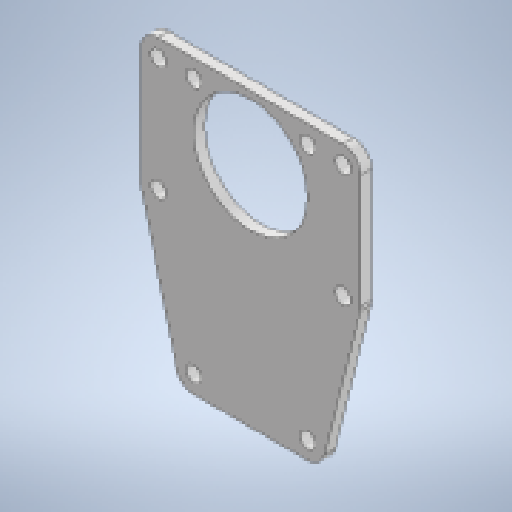
# Autodesk Inventor part: jouhansin_sita
Saved by Autodesk Inventor 2025.1 (Build 291241000, 241)
## iProperties
Created: 2024-09-01
Part Number: jouhansin_sita
Material: 一般
Document SubType Name: Modeling
Designer: right
Density: 1 g/cm^3
Appearance: 既定
Author: right
Autodesk Inventor part; units mm, degrees
ref_plane "YZ Plane" through (0, 0, 0) normal (1, 0, 0) x (0, 1, 0)
ref_plane "XZ Plane" through (0, 0, 0) normal (0, 1, 0) x (-1, 0, 0)
ref_plane "XY Plane" through (0, 0, 0) normal (0, 0, 1) x (1, 0, 0)
sketch "スケッチ1" plane through (0, 0, 0) normal (0, 0, 1) x (1, 0, 0)
  circle A0 centre (55.7151, -22.426) radius 1 projected
  circle A1 centre (55.7151, -6.426) radius 1.05 projected
  circle A2 centre (20.7151, -6.426) radius 1 projected
  circle A3 centre (4.7151, -6.426) radius 1.45 projected
  circle A4 centre (-30.2849, -22.426) radius 1 projected
  circle A5 centre (-30.2849, -6.426) radius 1.05 projected
  circle A6 centre (55.7151, -22.426) radius 1.1
  circle A7 centre (55.7151, -6.426) radius 1.1
  circle A8 centre (20.7151, -6.426) radius 1.1
  circle A9 centre (4.7151, -6.426) radius 1.1
  circle A10 centre (-30.2849, -6.426) radius 1.1
  circle A11 centre (-30.2849, -22.426) radius 1.1
  circle A12 centre (20.7151, -42.426) radius 1 projected
  circle A13 centre (4.7151, -42.426) radius 1 projected
  circle A14 centre (20.7151, -42.426) radius 1.1
  circle A15 centre (4.7151, -42.426) radius 1.1
  circle A16 centre (55.7151, -6.426) radius 2.5
  circle A17 centre (-30.2849, -6.426) radius 2.5
  circle A18 centre (-30.2849, -22.426) radius 2.5
  circle A19 centre (55.7151, -22.426) radius 2.5
  circle A20 centre (20.7151, -42.426) radius 2.5
  circle A21 centre (4.7151, -42.426) radius 2.5
  line L0 (21.9554, -44.5966) -> (56.9554, -24.5966)
  line L1 (58.2151, -22.426) -> (58.2151, -6.426)
  line L2 (55.7151, -3.926) -> (-30.2849, -3.926)
  line L3 (-32.7849, -6.426) -> (-32.7849, -22.426)
  line L4 (3.4747, -44.5966) -> (-31.5253, -24.5966)
  line L5 (20.7151, -44.926) -> (4.7151, -44.926)
  circle A22 centre (91.7151, -22.426) radius 1 projected
  circle A23 centre (91.7151, -22.426) radius 1.1
  circle A24 centre (-66.2849, -22.426) radius 1.05 projected
  circle A25 centre (-66.2849, -22.426) radius 1.1
  circle A26 centre (-66.2849, -22.426) radius 2.5
  circle A27 centre (91.7151, -22.426) radius 2.5
  line L6 (92.3929, -24.8324) -> (21.3929, -44.8324)
  line L7 (91.7151, -19.926) -> (55.7151, -19.926)
  line L8 (73.8937, -20.8546) -> (67.5365, -20.8546) projected
  line L9 (73.8937, -16.9974) -> (73.8937, -20.8546) projected
  line L10 (67.5365, -16.9974) -> (73.8937, -16.9974) projected
  line L11 (67.5365, -20.8546) -> (67.5365, -16.9974) projected
  line L12 (73.8937, -20.8546) -> (67.5365, -20.8546) projected
  line L13 (67.6151, -17.226) -> (73.6151, -17.226) projected
  line L14 (73.6151, -17.226) -> (73.6151, -20.726) projected
  line L15 (73.6151, -20.726) -> (67.6151, -20.726) projected
  line L16 (67.6151, -20.726) -> (67.6151, -17.226) projected
  line L17 (65.6151, -22.726) -> (75.6151, -22.726)
  line L18 (75.6151, -22.726) -> (75.6151, -15.226)
  line L19 (75.6151, -15.226) -> (65.6151, -15.226)
  line L20 (65.6151, -15.226) -> (65.6151, -22.726)
  line L21 (-66.9603, -24.833) -> (3.4747, -44.5966)
  line L22 (-30.2849, -19.926) -> (-66.2849, -19.926)
  line L23 (-48.4635, -20.8546) -> (-48.4635, -16.9974) projected
  line L24 (-28.7849, -24.426) -> (-67.7849, -24.426) projected
  arc A28 (-28.7849, -24.426) -> (-28.2849, -23.926) centre (-28.7849, -23.926) ccw projected
  line L25 (-28.2849, -4.926) -> (-28.2849, -23.926) projected
  arc A29 (-28.2849, -4.926) -> (-28.7849, -4.426) centre (-28.7849, -4.926) ccw projected
  line L26 (-67.7849, -4.426) -> (-28.7849, -4.426) projected
  arc A30 (-67.7849, -4.426) -> (-68.2849, -4.926) centre (-67.7849, -4.926) ccw projected
  line L27 (-68.2849, -23.926) -> (-68.2849, -4.926) projected
  arc A31 (-68.2849, -23.926) -> (-67.7849, -24.426) centre (-67.7849, -23.926) ccw projected
  line L28 (-48.4635, -7.9974) -> (-42.1063, -7.9974) projected
  line L29 (-42.1063, -7.9974) -> (-42.1063, -11.8546) projected
  line L30 (-42.1063, -11.8546) -> (-48.4635, -11.8546) projected
  line L31 (-48.4635, -11.8546) -> (-48.4635, -7.9974) projected
  circle A32 centre (-40.8849, -14.426) radius 1.1519 projected
  line L32 (-48.4635, -20.8546) -> (-48.4635, -16.9974) projected
  line L33 (-48.4635, -16.9974) -> (-42.1063, -16.9974) projected
  line L34 (-42.1063, -16.9974) -> (-42.1063, -20.8546) projected
  line L35 (-42.1063, -20.8546) -> (-48.4635, -20.8546) projected
  circle A33 centre (-66.2849, -6.426) radius 1.8131 projected
  circle A34 centre (-66.2849, -22.426) radius 1.8131 projected
  circle A35 centre (-30.2849, -6.426) radius 1.8131 projected
  circle A36 centre (-30.2849, -22.426) radius 1.8131 projected
  arc A37 (-59.7956, -8.176) -> (-59.7849, -20.676) centre (-59.7849, -14.426) ccw projected
  arc A38 (-60.0349, -7.926) -> (-59.7956, -8.1758) centre (-59.7849, -7.926) ccw projected
  line L36 (-60.0349, -7.926) -> (-60.0349, -6.176) projected
  arc A39 (-59.5349, -6.176) -> (-60.0349, -6.176) centre (-59.7849, -6.176) ccw projected
  line L37 (-59.5349, -6.176) -> (-59.5349, -7.926) projected
  arc A40 (-59.7849, -8.176) -> (-59.5349, -7.926) centre (-59.7849, -7.926) ccw projected
  arc A41 (-57.3931, -8.6518) -> (-59.7849, -8.176) centre (-59.7849, -14.426) ccw projected
  arc A42 (-57.5284, -8.3251) -> (-57.3931, -8.6518) centre (-57.2975, -8.4208) ccw projected
  line L38 (-57.5284, -8.3251) -> (-56.8587, -6.7083) projected
  arc A43 (-56.3968, -6.8997) -> (-56.8587, -6.7083) centre (-56.6278, -6.804) ccw projected
  line L39 (-56.3968, -6.8997) -> (-57.0665, -8.5165) projected
  arc A44 (-57.3931, -8.6518) -> (-57.0665, -8.5165) centre (-57.2975, -8.4208) ccw projected
  arc A45 (-55.3655, -10.0066) -> (-57.3931, -8.6518) centre (-59.7849, -14.426) ccw projected
  arc A46 (-55.3655, -9.653) -> (-55.3655, -10.0066) centre (-55.1887, -9.8298) ccw projected
  line L40 (-55.3655, -9.653) -> (-54.1281, -8.4156) projected
  arc A47 (-53.7745, -8.7692) -> (-54.1281, -8.4156) centre (-53.9513, -8.5924) ccw projected
  line L41 (-53.7745, -8.7692) -> (-55.0119, -10.0066) projected
  arc A48 (-55.3655, -10.0066) -> (-55.0119, -10.0066) centre (-55.1887, -9.8298) ccw projected
  arc A49 (-54.0107, -12.0342) -> (-55.3655, -10.0066) centre (-59.7849, -14.426) ccw projected
  arc A50 (-53.8754, -11.7076) -> (-54.0107, -12.0342) centre (-53.7797, -11.9386) ccw projected
  line L42 (-53.8754, -11.7076) -> (-52.2586, -11.0379) projected
  arc A51 (-52.0672, -11.4998) -> (-52.2586, -11.0379) centre (-52.1629, -11.2689) ccw projected
  line L43 (-52.0672, -11.4998) -> (-53.684, -12.1695) projected
  arc A52 (-54.0107, -12.0342) -> (-53.684, -12.1695) centre (-53.7797, -11.9386) ccw projected
  arc A53 (-53.5349, -14.426) -> (-54.0107, -12.0342) centre (-59.7849, -14.426) ccw projected
  arc A54 (-53.2849, -14.176) -> (-53.5349, -14.426) centre (-53.2849, -14.426) ccw projected
  line L44 (-53.2849, -14.176) -> (-51.5349, -14.176) projected
  arc A55 (-51.5349, -14.676) -> (-51.5349, -14.176) centre (-51.5349, -14.426) ccw projected
  line L45 (-51.5349, -14.676) -> (-53.2849, -14.676) projected
  arc A56 (-53.5349, -14.426) -> (-53.2849, -14.676) centre (-53.2849, -14.426) ccw projected
  arc A57 (-54.0107, -16.8178) -> (-53.5349, -14.426) centre (-59.7849, -14.426) ccw projected
  arc A58 (-53.684, -16.6825) -> (-54.0107, -16.8178) centre (-53.7797, -16.9134) ccw projected
  line L46 (-53.684, -16.6825) -> (-52.0672, -17.3522) projected
  arc A59 (-52.2586, -17.8141) -> (-52.0672, -17.3522) centre (-52.1629, -17.5831) ccw projected
  line L47 (-52.2586, -17.8141) -> (-53.8754, -17.1444) projected
  arc A60 (-54.0107, -16.8178) -> (-53.8754, -17.1444) centre (-53.7797, -16.9134) ccw projected
  arc A61 (-55.3655, -18.8454) -> (-54.0107, -16.8178) centre (-59.7849, -14.426) ccw projected
  arc A62 (-55.0119, -18.8454) -> (-55.3655, -18.8454) centre (-55.1887, -19.0222) ccw projected
  line L48 (-55.0119, -18.8454) -> (-53.7745, -20.0829) projected
  arc A63 (-54.1281, -20.4364) -> (-53.7745, -20.0829) centre (-53.9513, -20.2596) ccw projected
  line L49 (-54.1281, -20.4364) -> (-55.3655, -19.199) projected
  arc A64 (-55.3655, -18.8454) -> (-55.3655, -19.199) centre (-55.1887, -19.0222) ccw projected
  arc A65 (-57.3931, -20.2003) -> (-55.3655, -18.8454) centre (-59.7849, -14.426) ccw projected
  arc A66 (-57.0665, -20.3356) -> (-57.3931, -20.2003) centre (-57.2975, -20.4312) ccw projected
  line L50 (-57.0665, -20.3356) -> (-56.3968, -21.9523) projected
  arc A67 (-56.8587, -22.1437) -> (-56.3968, -21.9523) centre (-56.6278, -22.048) ccw projected
  line L51 (-56.8587, -22.1437) -> (-57.5284, -20.5269) projected
  arc A68 (-57.3931, -20.2003) -> (-57.5284, -20.5269) centre (-57.2975, -20.4312) ccw projected
  arc A69 (-59.7849, -20.676) -> (-57.3931, -20.2003) centre (-59.7849, -14.426) ccw projected
  arc A70 (-59.5349, -20.926) -> (-59.7849, -20.676) centre (-59.7849, -20.926) ccw projected
  line L52 (-59.5349, -20.926) -> (-59.5349, -22.676) projected
  arc A71 (-60.0349, -22.676) -> (-59.5349, -22.676) centre (-59.7849, -22.676) ccw projected
  line L53 (-60.0349, -22.676) -> (-60.0349, -20.926) projected
  arc A72 (-59.7849, -20.676) -> (-60.0349, -20.926) centre (-59.7849, -20.926) ccw projected
  line L54 (-50.4635, -22.8546) -> (-40.1063, -22.8546)
  line L55 (-40.1063, -22.8546) -> (-40.1063, -14.9974)
  line L56 (-40.1063, -14.9974) -> (-50.4635, -14.9974)
  line L57 (-50.4635, -22.8546) -> (-50.4635, -14.9974)
  circle A73 centre (-59.7849, -14.426) radius 8 projected
  circle A74 centre (85.2151, -14.426) radius 8 projected
  point P0 (0, 0)
  point P1 (-32.7849, -19.926)
  point P2 (-40.1063, -19.926)
  point P3 (-50.4635, -19.926)
  point P4 (-53.9314, -19.926)
  point P5 (-54.3076, -20.2569)
  point P6 (-56.494, -21.7178)
  point P7 (-56.9559, -21.9091)
  point P8 (-59.5349, -22.4221)
  point P9 (-60.0349, -22.4221)
  point P10 (-65.4578, -20.0668)
  point P11 (65.6151, -19.926)
  point P12 (58.2151, -19.926)
  point P13 (90.888, -20.0668)
  point P14 (79.4056, -19.926)
  point P15 (75.6151, -19.926)
  dimension "d0" = 2.2
  dimension "d1" = 2.2
  dimension "d2" = 2.2
  dimension "d3" = 2.2
  dimension "d4" = 2.2
  dimension "d5" = 2.2
  dimension "d6" = 2.2
  dimension "d7" = 2.2
  dimension "d8" = 5
  dimension "d9" = 5
  dimension "d10" = 5
  dimension "d11" = 5
  dimension "d12" = 5
  dimension "d13" = 5
  dimension "d18" = 2.2
  dimension "d19" = 2.2
  dimension "d20" = 5
  dimension "d21" = 5
  dimension "d22" = 2
  dimension "d23" = 2
  dimension "d24" = 2
  constraints: 36 end point, 19 point on circle, 19 tangent, 18 centre point, 18 coincident, 1 parallel, 5 other
  measures "d0" diameter of A6
  measures "d1" diameter of A7
  measures "d2" diameter of A8
  measures "d3" diameter of A9
  measures "d4" diameter of A10
  measures "d5" diameter of A11
  measures "d6" diameter of A14
  measures "d7" diameter of A15
  measures "d8" diameter of A16
  measures "d9" diameter of A17
  measures "d10" diameter of A18
  measures "d11" diameter of A19
  measures "d12" diameter of A20
  measures "d13" diameter of A21
  measures "d18" diameter of A23
  measures "d19" diameter of A25
  measures "d20" diameter of A26
  measures "d21" diameter of A27
  measures "d22" distance between parallel lines of L15 L17
  measures "d23" distance between parallel lines of L35 L54
  measures "d24" distance between parallel lines of L23 L57
extrude "押し出し1" add sketch "スケッチ1" along normal blind 1.5 contours A3 | A16 | L1 L7 A19 L0 A20 L5 A21 L4 A18 A28 L25 A17 A29 L2 A16 | L7 L20 L17 L18 A74 A27 L6 A20 L0 A19 L1 | L1 A19 L7 | A17 L26 | A19 | A29 A17 | A17 L25 L26 | A17 L25 | A17 L25 A18 L22 L3 | A20 | L22 A18 L3 | L3 A18 L24 A26 A73 L53 A71 L52 L51 A67 L50 L49 A63 L48 L22 L57 L54 L55 | L25 A18 L24 | A18 L25 | L27 A26 | A26 A73 L24 L27 | A27 A74 | A28 A18 | L24 A18 | A18 L4 L21 A26 L24 | A21 | A26 L24 | A34 | A35 | A36 picked at (89.8821, -21.5749)
sketch "スケッチ2" plane through (0, 0, 1.5) normal (0, 0, 1) x (1, 0, 0)
  circle A0 centre (12.7151, -12.926) radius 8 projected
  point P0 (0, 0)
extrude "押し出し2" cut sketch "スケッチ2" against normal through all
fillet "フィレット1" radius 2 8 edges at (75.6151, -19.926, 0.75) (75.6151, -22.726, 0.75) (65.6151, -22.726, 0.75) (65.6151, -19.926, 0.75) (-50.4635, -19.926, 0.75) (-50.4635, -22.8546, 0.75) (-40.1063, -22.8546, 0.75) (-40.1063, -19.926, 0.75)
